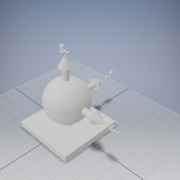
# Autodesk Inventor part: center-piece
Saved by Autodesk Inventor 2018 (Build 220112000, 112)
## iProperties
Created: 2018-03-12
Part Number: center-piece
Material: Generic
Document SubType Name: Modeling
Designer: Unknown6656
Density: 1 g/cm^3
Appearance: Default
Mass: 292121 g
Surface Area: 44589.4 cm^2
Volume: 292121 cm^3
Author: Unknown6656
Autodesk Inventor part; units mm, degrees
ref_plane "YZ Plane" through (0, 0, 0) normal (1, 0, 0) x (0, 1, 0)
ref_plane "XZ Plane" through (0, 0, 0) normal (0, 1, 0) x (-1, 0, 0)
ref_plane "XY Plane" through (0, 0, 0) normal (0, 0, 1) x (1, 0, 0)
sketch "Sketch1" plane through (0, 0, 0) normal (0, 0, 1) x (1, 0, 0)
  line L0 (-500, -500) -> (500, -500)
  line L1 (500, -500) -> (500, 500)
  line L2 (500, 500) -> (-500, 500)
  line L3 (-500, 500) -> (-500, -500)
  line L4 (-500, -500) -> (500, 500) construction
  line L5 (500, -500) -> (-500, 500) construction
  point P0 (0, 0)
  dimension "d0" = 1000
  dimension "d1" = 1000
  constraints: 12 end point, 2 midpoint, 2 parallel, 1 horizontal, 1 perpendicular
  measures "d0" distance of L2.end L1.end
  measures "d1" distance of L1.end L0.end
extrude "Extrusion1" add sketch "Sketch1" along normal blind 100
sketch "Sketch2" plane through (0, 0, 0) normal (0, 1, 0) x (-1, 0, 0)
  line L0 (0, 0) -> (0, 500)
  line L1 (0, 0) -> (100, 0)
  line L2 (100, 0) -> (100, 164.5898)
  line L3 (0, 500) -> (0, 850)
  arc A0 (100, 164.5898) -> (0, 850) centre (0, 500) ccw
  dimension "d4" = 500
  dimension "d5" = 100
  dimension "d6" = 350
  constraints: 8 end point, 2 point on circle, 2 vertical, 1 centre point, 1 coincident, 1 horizontal, 1 perpendicular
  measures "d4" distance of L0.start L0.end
  measures "d5" distance of L0.start L1.end
  measures "d6" distance of L0.end L3.end
revolve "Revolution1" add sketch "Sketch2" angle 360 about axis through (0, 0, 0) along (0, 0, 1)
sketch "Sketch3" plane through (0, 0, 0) normal (1, 0, 0) x (0, 1, 0)
  line L0 (0, -170) -> (0, 1020) projected
  line L1 (0, 500) -> (-50, 500)
  line L2 (-50, 500) -> (-50, 1050)
  line L3 (-50, 1050) -> (-100, 1050)
  line L4 (-100, 1050) -> (0, 1223.2051)
  line L5 (0, 500) -> (0, 1223.2051)
  point P0 (0, 0)
  dimension "d8" = 500
  dimension "d9" = 50
  dimension "d10" = 550
  dimension "d11" = 30
  dimension "d12" = 50
  constraints: 10 end point, 3 perpendicular, 2 point on line, 1 horizontal
  measures "d8" distance from line of point (0, 0) L1
  measures "d9" distance between parallel lines of L0 L2
  measures "d10" distance of L1.end L2.end
  measures "d11" angle of L5 L4
  measures "d12" distance of L2.end L3.end
revolve "Revolution2" add sketch "Sketch3" angle 360 about axis through (0, 0, -10) along (0, 0, 1)
ref_plane "Work Plane1" through (0, 0, 500) normal (0, 0, -1) x (-1, 0, 0)
pattern_circular "Circular Pattern1" count 2 over 90 about axis through (0, 0, 500) along (0, 1, 0) of "Revolution2"
pattern_circular "Circular Pattern2" count 2 over 90 about axis through (0, 0, 500) along (-1, 0, 0) of "Revolution2"
sketch "Sketch4" plane through (0, 0, 0) normal (0, 1, 0) x (-1, 0, 0)
  circle A0 centre (0, 500) radius 50 projected
  line L0 (-346.4102, 450) -> (-346.4102, 550) projected
  line L1 (-50, 846.4102) -> (50, 846.4102) projected
  line L2 (-100, 164.5898) -> (100, 164.5898) projected
  line L3 (-550, 600) -> (-550, 400) projected
  line L4 (50, 1050) -> (-50, 1050) projected
  line L5 (-50, 846.4102) -> (50, 846.4102) projected
  line L6 (744.641, 500) -> (-967.8461, 500) projected
  line L7 (0, -244.641) -> (0, 1467.8461) projected
  line L8 (-963.1346, 560.6641) -> (-790.7331, 560.6641) construction
  line L9 (-790.7331, 560.6641) -> (-790.7331, 460.6641) construction
  line L10 (-790.7331, 460.6641) -> (-963.1346, 460.6641) construction
  line L11 (-963.1346, 460.6641) -> (-963.1346, 560.6641) construction
  line L12 (-85.6228, 1342.8567) -> (86.7786, 1342.8567) construction
  line L13 (86.7786, 1342.8567) -> (86.7786, 1242.8567) construction
  line L14 (86.7786, 1242.8567) -> (-85.6228, 1242.8567) construction
  line L15 (-85.6228, 1242.8567) -> (-85.6228, 1342.8567) construction
  line L16 (-5.7841, 1278.7886) -> (-35.8917, 1278.7886)
  line L17 (-35.8917, 1278.7886) -> (-35.8917, 1247.6058)
  line L18 (-35.8917, 1247.6058) -> (-49.0637, 1247.6058)
  line L19 (-49.0637, 1247.6058) -> (-49.0637, 1278.7886)
  line L20 (-49.0637, 1278.7886) -> (-79.1712, 1278.7886)
  line L21 (-79.1712, 1278.7886) -> (-79.1712, 1290.4373)
  line L22 (-79.1712, 1290.4373) -> (-49.0637, 1290.4373)
  line L23 (-49.0637, 1290.4373) -> (-49.0637, 1321.4409)
  line L24 (-49.0637, 1321.4409) -> (-35.8917, 1321.4409)
  line L25 (-35.8917, 1321.4409) -> (-35.8917, 1290.4373)
  line L26 (-35.8917, 1290.4373) -> (-5.7841, 1290.4373)
  line L27 (-5.7841, 1290.4373) -> (-5.7841, 1278.7886)
  line L28 (77.1908, 1332.1936) -> (26.1155, 1255.5807)
  line L29 (26.1155, 1255.5807) -> (78.1764, 1255.5807)
  line L30 (78.1764, 1255.5807) -> (78.1764, 1242.8567)
  line L31 (78.1764, 1242.8567) -> (9.0904, 1242.8567)
  line L32 (9.0904, 1242.8567) -> (9.0904, 1252.9821)
  line L33 (9.0904, 1252.9821) -> (60.4345, 1330.4911)
  line L34 (60.4345, 1330.4911) -> (10.4345, 1330.4911)
  line L35 (10.4345, 1330.4911) -> (10.4345, 1342.8567)
  line L36 (10.4345, 1342.8567) -> (77.1908, 1342.8567)
  line L37 (77.1908, 1342.8567) -> (77.1908, 1332.1936)
  line L38 (-883.2959, 496.596) -> (-913.4034, 496.596)
  line L39 (-913.4034, 496.596) -> (-913.4034, 465.4132)
  line L40 (-913.4034, 465.4132) -> (-926.5754, 465.4132)
  line L41 (-926.5754, 465.4132) -> (-926.5754, 496.596)
  line L42 (-926.5754, 496.596) -> (-956.683, 496.596)
  line L43 (-956.683, 496.596) -> (-956.683, 508.2447)
  line L44 (-956.683, 508.2447) -> (-926.5754, 508.2447)
  line L45 (-926.5754, 508.2447) -> (-926.5754, 539.2483)
  line L46 (-926.5754, 539.2483) -> (-913.4034, 539.2483)
  line L47 (-913.4034, 539.2483) -> (-913.4034, 508.2447)
  line L48 (-913.4034, 508.2447) -> (-883.2959, 508.2447)
  line L49 (-883.2959, 508.2447) -> (-883.2959, 496.596)
  line L50 (-792.6149, 460.6641) -> (-809.8192, 460.6641)
  line L51 (-809.8192, 460.6641) -> (-834.1023, 499.1945)
  line L52 (-834.1023, 499.1945) -> (-858.5647, 460.6641)
  line L53 (-858.5647, 460.6641) -> (-875.5898, 460.6641)
  line L54 (-875.5898, 460.6641) -> (-842.2564, 512.0978)
  line L55 (-842.2564, 512.0978) -> (-872.9016, 560.6641)
  line L56 (-872.9016, 560.6641) -> (-856.7726, 560.6641)
  line L57 (-856.7726, 560.6641) -> (-833.9231, 525.001)
  line L58 (-833.9231, 525.001) -> (-810.8048, 560.6641)
  line L59 (-810.8048, 560.6641) -> (-795.1238, 560.6641)
  line L60 (-795.1238, 560.6641) -> (-825.769, 512.3666)
  line L61 (-825.769, 512.3666) -> (-792.6149, 460.6641)
  point P0 (0, 0)
  point P1 (-723.2051, 500)
  constraints: 4 other
extrude "Extrusion2" add sketch "Sketch4" along normal mid plane 40 contours L49 L38 L39 L40 L41 L42 L43 L6 | L6 L43 L44 L45 L46 L47 L48 L49 | L61 L50 L51 L52 L53 L54 L6 | L6 L54 L55 L56 L57 L58 L59 L60 L61 | L16 L17 L18 L19 L20 L21 L22 L23 L24 L25 L26 L27 | L28 L29 L30 L31 L32 L33 L34 L35 L36 L37
sketch "Sketch5" plane through (0, 0, 0) normal (1, 0, 0) x (0, 1, 0)
  line L0 (346.4102, 550) -> (346.4102, 450) projected
  circle A0 centre (0, 500) radius 50 projected
  line L1 (-50, 846.4102) -> (50, 846.4102) projected
  line L2 (-100, 164.5898) -> (100, 164.5898) projected
  line L3 (550, 400) -> (550, 600) projected
  line L4 (100, 1050) -> (-100, 1050) projected
  line L5 (0, -268.5713) -> (0, 1611.428) projected
  line L6 (-744.641, 500) -> (967.8461, 500) projected
  line L7 (787.1297, 563.065) -> (959.5311, 563.065) construction
  line L8 (959.5311, 563.065) -> (959.5311, 463.065) construction
  line L9 (959.5311, 463.065) -> (787.1297, 463.065) construction
  line L10 (787.1297, 463.065) -> (787.1297, 563.065) construction
  line L11 (866.9684, 498.9969) -> (836.8608, 498.9969)
  line L12 (836.8608, 498.9969) -> (836.8608, 467.8141)
  line L13 (836.8608, 467.8141) -> (823.6888, 467.8141)
  line L14 (823.6888, 467.8141) -> (823.6888, 498.9969)
  line L15 (823.6888, 498.9969) -> (793.5813, 498.9969)
  line L16 (793.5813, 498.9969) -> (793.5813, 510.6456)
  line L17 (793.5813, 510.6456) -> (823.6888, 510.6456)
  line L18 (823.6888, 510.6456) -> (823.6888, 541.6492)
  line L19 (823.6888, 541.6492) -> (836.8608, 541.6492)
  line L20 (836.8608, 541.6492) -> (836.8608, 510.6456)
  line L21 (836.8608, 510.6456) -> (866.9684, 510.6456)
  line L22 (866.9684, 510.6456) -> (866.9684, 498.9969)
  line L23 (959.5311, 563.065) -> (923.3304, 498.8177)
  line L24 (923.3304, 498.8177) -> (923.3304, 463.065)
  line L25 (923.3304, 463.065) -> (909.5311, 463.065)
  line L26 (909.5311, 463.065) -> (909.5311, 499.0865)
  line L27 (909.5311, 499.0865) -> (873.3304, 563.065)
  line L28 (873.3304, 563.065) -> (889.8178, 563.065)
  line L29 (889.8178, 563.065) -> (909.7103, 526.5058)
  line L30 (909.7103, 526.5058) -> (917.058, 511.8105)
  line L31 (917.058, 511.8105) -> (923.7784, 525.0722)
  line L32 (923.7784, 525.0722) -> (943.9397, 563.065)
  line L33 (943.9397, 563.065) -> (959.5311, 563.065)
  point P0 (0, 0)
  point P1 (723.2051, 500)
  point P2 (0, 1223.2051)
  constraints: 2 other
extrude "Extrusion3" add sketch "Sketch5" along normal mid plane 40 contours L27 L28 L29 L30 L31 L32 L33 L23 L6 | L6 L23 L24 L25 L26 L27 | L16 L17 L18 L19 L20 L21 L22 L6 | L6 L22 L11 L12 L13 L14 L15 L16
body "Solid1"
